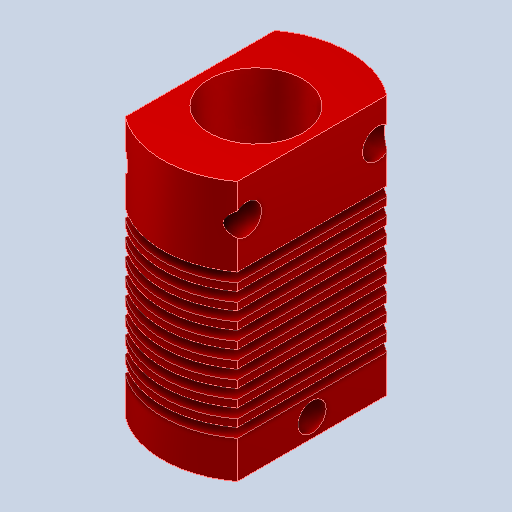
# Autodesk Inventor part: ENDER 3 RAD
Saved by Autodesk Inventor 2022 (Build 260153070, 153G)
## iProperties
Created: 2022-01-01
Part Number: ENDER 3 RAD
Material: Aluminum 6061
Document SubType Name: Modeling
Designer: a laptop
Density: 2.7 g/cm^3
Appearance: Aluminum - Flat
Author: a laptop
Autodesk Inventor part; units mm, degrees
ref_plane "YZ Plane" through (0, 0, 0) normal (1, 0, 0) x (0, 1, 0)
ref_plane "XZ Plane" through (0, 0, 0) normal (0, 1, 0) x (-1, 0, 0)
sketch "Sketch1" plane through (0, 0, 0) normal (0, 1, 0) x (-1, 0, 0)
  line L0 (6, 8) -> (6, -8)
  line L1 (-6, 8) -> (-6, -8)
  arc A0 (6, 8) -> (-6, 8) centre (0, 0) ccw
  arc A1 (-6, -8) -> (6, -8) centre (0, 0) ccw
  circle A2 centre (1.5, 7) radius 1.5
  line L2 (0, 0) -> (6, 0) construction
  circle A3 centre (1.5, -7) radius 1.5
  circle A4 centre (0, 0) radius 3.5
  circle A5 centre (0, 0) radius 4.3
  dimension "d0" = 10
  dimension "d1" = 10
  dimension "d3" = 12
  dimension "d4" = 3
  dimension "d5" = 7
  dimension "d6" = 1.5
  dimension "d7" = 7
  dimension "d16" = 8.6
  constraints: 6 centre point, 6 end point, 4 coincident, 4 point on circle, 2 vertical, 1 horizontal alignment, 1 parallel, 1 perpendicular, 1 symmetric about line, 1 other
  measures "d0" radius of A0
  measures "d1" radius of A1
  measures "d3" distance between parallel lines of L1 L0
  measures "d4" diameter of A2
  measures "d5" vertical distance of point (0, 0) A2.centre
  measures "d6" horizontal distance of point (0, 0) A2.centre
  measures "d7" diameter of A4
  measures "d16" diameter of A5
extrude "Extrusion1" add sketch "Sketch1" along normal blind 27.8 contours L0 A1 L1 A0 | A2 | A3 | A5
ref_plane "Work Plane1" through (0, 4, 0) normal (0, -1, 0) x (1, 0, 0)
sketch "Sketch2" plane through (0, 4, 0) normal (0, -1, 0) x (1, 0, 0)
  line L0 (-6, -8) -> (-6, 8) projected
  arc A0 (6, 8) -> (-6, 8) centre (0, 0) ccw projected
  line L1 (6, 8) -> (6, -8) projected
  arc A1 (-6, -8) -> (6, -8) centre (0, 0) ccw projected
extrude "Extrusion2" cut sketch "Sketch2" against normal blind 1
pattern_linear "Rectangular Pattern1" count 9 spacing 1.8 along (0, 1, 0) of "Extrusion2"
extrude "Extrusion3" add sketch "Sketch1" along normal blind 16.7 contours A5
sketch "Sketch3" plane through (0, 16.7, 0) normal (0, 1, 0) x (1, 0, 0)
  circle A0 centre (0, 0) radius 4.3 projected
  circle A1 centre (0, 0) radius 3
  dimension "d19" = 6
  constraints: 1 centre point, 1 coincident
  measures "d19" diameter of A1
extrude "Extrusion4" add sketch "Sketch3" along normal blind 3.1
sketch "Sketch4" plane through (0, 27.8, 0) normal (0, 1, 0) x (1, 0, 0)
  circle A0 centre (0, 0) radius 5
  dimension "d22" = 10
  constraints: 1 centre point, 1 coincident
  measures "d22" diameter of A0
extrude "Extrusion5" cut sketch "Sketch4" against normal blind 8
extrude "Extrusion6" cut sketch "Sketch1" along normal blind 4 contours A2 | A3
sketch "Sketch5" plane through (6, 27.8, 8) normal (1, 0, 0) x (0, 0, -1)
  circle A0 centre (1, -4) radius 1.6
  circle A1 centre (15, -4) radius 1.6
  point P0 (8, -27.8)
  dimension "d27" = 3.2
  dimension "d28" = 23.8
  dimension "d29" = 14
  dimension "d31" = 7
  constraints: 2 centre point, 1 equal radius, 1 horizontal alignment
  measures "d27" diameter of A1
  measures "d28" vertical distance of A1.centre point (8, -27.8)
  measures "d29" distance of A1.centre A0.centre
  measures "d31" horizontal distance of point (8, -27.8) A1.centre
extrude "Extrusion7" cut sketch "Sketch5" against normal blind 12
sketch "Sketch6" plane through (6, 0, 8) normal (1, 0, 0) x (0, 0, -1)
  circle A0 centre (8, 2) radius 1.5
  line L0 (0, 0) -> (16, 0) projected
  point P0 (8, 0)
  point P1 (8, 0)
  dimension "d34" = 2
  dimension "d35" = 3
  constraints: 1 centre point, 1 midpoint, 1 vertical alignment
  measures "d34" distance of A0.centre point (8, 0)
  measures "d35" diameter of A0
extrude "Extrusion8" cut sketch "Sketch6" against normal blind 4.75
body "Solid1"
